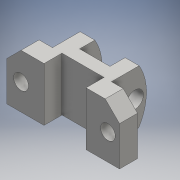
# Autodesk Inventor part: 240510_3Dsketch07
Saved by Autodesk Inventor 2016 (Build 200138000, 138)
## iProperties
Created: 2024-05-10
Part Number: 240510_3Dsketch07
Material: 일반
Document SubType Name: Modeling
Designer: pc
Density: 1 g/cm^3
Appearance: 기본값
Author: pc
Autodesk Inventor part; units mm, degrees
ref_plane "YZ Plane" through (0, 0, 0) normal (1, 0, 0) x (0, 1, 0)
ref_plane "XZ Plane" through (0, 0, 0) normal (0, 1, 0) x (-1, 0, 0)
ref_plane "XY Plane" through (0, 0, 0) normal (0, 0, 1) x (1, 0, 0)
sketch "스케치1" plane through (0, 0, 0) normal (0, 0, 1) x (1, 0, 0)
  line L0 (31.5724, -15.0322) -> (-31.5724, -15.0322)
  line L1 (-31.5724, -15.0322) -> (-31.5724, 15.0322)
  line L2 (-31.5724, 15.0322) -> (31.5724, 15.0322)
  line L3 (31.5724, 15.0322) -> (31.5724, -15.0322)
  line L4 (31.5724, -15.0322) -> (-31.5724, 15.0322) construction
  line L5 (-31.5724, -15.0322) -> (31.5724, 15.0322) construction
  point P0 (0, 0)
  constraints: 12 end point, 2 midpoint, 2 parallel, 1 horizontal, 1 perpendicular
extrude "돌출1" add sketch "스케치1" along normal blind 30
sketch "스케치2" plane through (-31.5724, 15.0322, 0) normal (0, 1, 0) x (1, 0, 0)
  point P0 (31.5724, 0)
sketch "스케치3" plane through (-31.5724, 15.0322, 0) normal (0, 1, 0) x (1, 0, 0)
  line L0 (63.1447, 0) -> (0, 0) projected
  line L1 (15.5145, 0) -> (15.5145, -30)
  line L2 (0, -30) -> (63.1447, -30) projected
  line L3 (48.5426, 0) -> (48.5426, -30)
  line L4 (63.1447, -30) -> (0, -30) projected
  line L5 (15.5145, -30) -> (0, -30)
  line L6 (0, 0) -> (63.1447, 0) projected
  line L7 (0, -30) -> (0, 0)
  line L8 (0, 0) -> (15.5145, 0)
  line L9 (48.5426, 0) -> (63.1447, 0)
  line L10 (63.1447, 0) -> (63.1447, -30)
  line L11 (63.1447, -30) -> (48.5426, -30)
  line L12 (23.7136, 0) -> (40.7128, 0)
  line L13 (40.7128, 0) -> (40.7128, -30)
  line L14 (40.7128, -30) -> (23.7136, -30)
  line L15 (23.7136, -30) -> (23.7136, 0)
  point P0 (31.5724, 0)
  constraints: 24 end point, 6 point on line, 4 perpendicular, 3 parallel, 2 collinear, 2 horizontal, 1 vertical
extrude "돌출2" cut sketch "스케치3" against normal blind 20 contours L10 L2 L3 L0 | L1 L2 L7 L0
extrude "돌출3" cut sketch "스케치3" against normal blind 13 contours L13 L2 L15 L0
sketch "스케치4" plane through (0, 0, 30) normal (0, 0, 1) x (1, 0, 0)
  line L0 (-31.5724, -15.0322) -> (31.5724, -15.0322) projected
  line L1 (-10.7158, -4.9678) -> (12.8298, -4.9678)
  line L2 (12.8298, -4.9678) -> (12.8298, -15.0322)
  line L3 (12.8298, -15.0322) -> (-10.7158, -15.0322)
  line L4 (-10.7158, -15.0322) -> (-10.7158, -4.9678)
  point P0 (0, 0)
  constraints: 8 end point, 2 parallel, 1 horizontal, 1 perpendicular, 1 point on line
extrude "돌출4" cut sketch "스케치4" against normal blind 50
sketch "스케치5" plane through (16.9702, 15.0322, 30) normal (1, 0, 0) x (0, 0, -1)
  circle A0 centre (15.2748, -6.7584) radius 4.7017
  point P0 (30, -15.0322)
  constraints: 1 centre point
extrude "돌출5" cut sketch "스케치5" against normal blind 50
sketch "스케치6" plane through (-31.5724, -4.9678, 0) normal (0, 1, 0) x (1, 0, 0)
  circle A0 centre (56.6423, -14.736) radius 4.1041
  circle A1 centre (7.9978, -14.736) radius 4.1777
  point P0 (31.5724, 0)
  constraints: 2 centre point
extrude "돌출6" cut sketch "스케치6" against normal blind 50
chamfer "모따기1" distance 8 angle 45 2 edges at (-31.5724, -10, 30) (31.5724, -10, 30)
sketch "스케치7" plane through (16.9702, 15.0322, 30) normal (1, 0, 0) x (0, 0, -1)
  point P0 (30, -15.0322)
sketch "스케치8" plane through (16.9702, 15.0322, 30) normal (1, 0, 0) x (0, 0, -1)
  line L0 (30, 0) -> (30, -20) projected
  line L1 (0, 0) -> (0, -13) projected
  arc A0 (30, -4.7173) -> (0, -4.4986) centre (14.8208, -29.1901) ccw
  line L2 (0, -4.4986) -> (0, 0)
  line L3 (0, 0) -> (30, 0) projected
  line L4 (30, 0) -> (30, -4.7173)
  point P0 (30, -15.0322)
  constraints: 4 end point, 2 collinear, 2 point on circle, 2 point on line, 1 centre point
extrude "돌출7" cut sketch "스케치8" against normal blind 50
